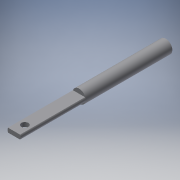
# Autodesk Inventor part: Ring Connector model
Saved by Autodesk Inventor 2017 (Build 210142000, 142)
## iProperties
Created: 2017-03-02
Part Number: Ring Connector model
Material: Generic
Document SubType Name: Modeling
Designer: coffmant
Density: 1 g/cm^3
Appearance: Default
Quantity: 1
Author: coffmant
Autodesk Inventor part; units mm, degrees
ref_plane "YZ Plane" through (0, 0, 0) normal (1, 0, 0) x (0, 1, 0)
ref_plane "XZ Plane" through (0, 0, 0) normal (0, 1, 0) x (-1, 0, 0)
ref_plane "XY Plane" through (0, 0, 0) normal (0, 0, 1) x (1, 0, 0)
sketch "Sketch1" plane through (0, 0, 0) normal (0, 0, 1) x (1, 0, 0)
  circle A0 centre (0, 0) radius 7.747
  dimension "d0" = 15.494
  constraints: 1 centre point, 1 coincident
  measures "d0" diameter of A0
extrude "Extrusion1" add sketch "Sketch1" along normal blind 101.6
sketch "Sketch2" plane through (0, 0, 101.6) normal (0, 0, 1) x (1, 0, 0)
  line L0 (-7.3325, 2.5) -> (6.8096, 2.5)
  line L1 (-7.3325, -2.5) -> (6.8096, -2.5)
  arc A0 (-7.3325, 2.5) -> (-7.3325, -2.5) centre (-4.4675, 0) ccw
  arc A1 (6.8096, -2.5) -> (6.8096, 2.5) centre (3.9446, 0) ccw
  circle A2 centre (0, 0) radius 7.747 projected
  point P0 (7.747, 0)
  dimension "d3" = 2.5
  dimension "d4" = 2.5
  dimension "d5" = 14.1421
  dimension "d6" = 14.1421
  constraints: 8 point on circle, 4 end point, 2 centre point, 1 equal radius, 1 horizontal, 1 parallel
  measures "d3" distance from line of point (0, 0) L0
  measures "d4" distance from line of point (0, 0) L1
  measures "d5" distance of L0.end L0.start
  measures "d6" distance of L1.start L1.end
extrude "Extrusion2" add sketch "Sketch2" along normal blind 76.2 contours L0 A1 L1 A2
sketch "Sketch3" plane through (-7.3325, 2.5, 101.6) normal (0, 1, 0) x (1, 0, 0)
  circle A0 centre (7.0711, -63.5) radius 4.1021
  line L0 (14.1421, -76.2) -> (0, -76.2) projected
  line L1 (0, 0) -> (0, -76.2) projected
  line L2 (14.1421, 0) -> (14.1421, -76.2) projected
  point P0 (7.3325, 101.6)
  dimension "d9" = 8.2042
  dimension "d10" = 12.7
  dimension "d11" = 7.0711
  dimension "d12" = 14.1421
  constraints: 1 centre point
  measures "d9" diameter of A0
  measures "d10" distance from line of L0 A0.centre
  measures "d11" distance from line of L1 A0.centre
  measures "d12" distance between parallel lines of L2 L1
extrude "Extrusion3" cut sketch "Sketch3" against normal through all
equation "\"d4\" = d3"
equation "\"d11\" = 0.5 * d12"
body "Solid1"
